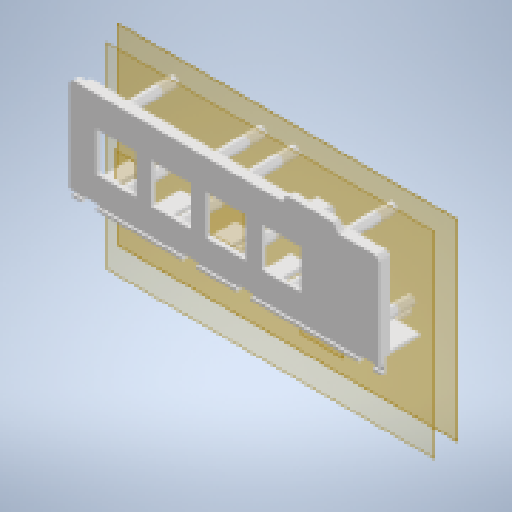
# Autodesk Inventor part: RV_ES_TopHV
Saved by Autodesk Inventor 2024.2 (Build 282272000, 272)
## iProperties
Created: 2023-08-06
Part Number: RV_ES_TopHV
Material: Generic
Document SubType Name: Modeling
Designer: atrus
Density: 1 g/cm^3
Appearance: Default
Mass: 78.5507 g
Surface Area: 462.891 cm^2
Volume: 78.5507 cm^3
Author: atrus
Autodesk Inventor part; units mm, degrees
ref_plane "YZ Plane" through (0, 0, 0) normal (1, 0, 0) x (0, 1, 0)
ref_plane "XZ Plane" through (0, 0, 0) normal (0, 1, 0) x (-1, 0, 0)
ref_plane "Work Plane1" through (160.7185, -7.942384, -39.091557) normal (0, 0, 1) x (1, 0, 0)
ref_plane "Bottom Case Offset" through (160.7185, -7.942384, -38.891557) normal (0, 0, 1) x (1, 0, 0)
sketch "Sketch1" plane through (0, 0, 0) normal (0, 0, 1) x (1, 0, 0)
  line L0 (0, 55.614096) -> (215.9, 55.614096)
  line L1 (215.9, 55.614096) -> (215.9, 121.724616)
  line L2 (215.9, 121.724616) -> (0, 121.724616)
  line L3 (0, 121.724616) -> (0, 55.614096)
  line L4 (215.9, 121.724616) -> (215.9, 57.656276) construction
  line L5 (0, 48.884616) -> (0, 118.549616)
  line L6 (1.113, 48.884616) -> (0, 48.884616)
  point P0 (0, 88.669356)
  constraints: 10 end point, 2 parallel, 1 horizontal, 1 midpoint, 1 perpendicular
extrude "Top Face" add sketch "Sketch1" along normal blind 5
sketch "Sketch2" plane through (0, 0, 5) normal (0, 0, 1) x (1, 0, 0)
  line L0 (44.754719, 74.175735) -> (19.253119, 74.175735) construction
  line L1 (44.754719, 99.677335) -> (44.754719, 74.175735) construction
  line L2 (19.253119, 74.175735) -> (19.253119, 99.677335) construction
  line L3 (57.607119, 74.175735) -> (57.607119, 99.677335) construction
  line L4 (83.108719, 99.677335) -> (83.108719, 74.175735) construction
  line L5 (83.108719, 74.175735) -> (57.607119, 74.175735) construction
  line L6 (96.215119, 74.175735) -> (96.215119, 99.677335) construction
  line L7 (121.716719, 99.677335) -> (121.716719, 74.175735) construction
  line L8 (134.823119, 74.175735) -> (134.823119, 99.677335) construction
  line L9 (160.324719, 99.677335) -> (160.324719, 74.175735) construction
  line L10 (160.324719, 74.175735) -> (134.823119, 74.175735) construction
  line L11 (19.253119, 99.677335) -> (44.754719, 99.677335) construction
  line L12 (57.607119, 99.677335) -> (83.108719, 99.677335) construction
  line L13 (96.215119, 99.677335) -> (121.716719, 99.677335) construction
  line L14 (134.823119, 99.677335) -> (160.324719, 99.677335) construction
  line L15 (18.253119, 100.677335) -> (18.253119, 73.175735)
  line L16 (18.253119, 73.175735) -> (45.754719, 73.175735)
  line L17 (45.754719, 73.175735) -> (45.754719, 100.677335)
  line L18 (45.754719, 100.677335) -> (18.253119, 100.677335)
  line L19 (56.607119, 100.677335) -> (56.607119, 73.175735)
  line L20 (56.607119, 73.175735) -> (84.108719, 73.175735)
  line L21 (84.108719, 73.175735) -> (84.108719, 100.677335)
  line L22 (84.108719, 100.677335) -> (56.607119, 100.677335)
  line L23 (121.716719, 74.175735) -> (96.215119, 74.175735) construction
  line L24 (96.215119, 74.175735) -> (96.215119, 99.677335)
  line L25 (95.215119, 100.677335) -> (95.215119, 73.175735)
  line L26 (95.215119, 73.175735) -> (122.716719, 73.175735)
  line L27 (122.716719, 73.175735) -> (122.716719, 100.677335)
  line L28 (122.716719, 100.677335) -> (95.215119, 100.677335)
  line L29 (133.823119, 100.677335) -> (133.823119, 73.175735)
  line L30 (133.823119, 73.175735) -> (161.324719, 73.175735)
  line L31 (161.324719, 73.175735) -> (161.324719, 100.677335)
  line L32 (161.324719, 100.677335) -> (133.823119, 100.677335)
  point P0 (0, 0)
  dimension "d96" = 1
  constraints: 32 end point, 3 parallel, 12 other
  measures "d96" distance between parallel lines of L18 L11
extrude "Recept Cutouts" cut sketch "Sketch2" against normal blind 3
sketch "Sketch3" plane through (0, 0, 0) normal (0, 0, -1) x (-1, 0, 0)
  circle A0 centre (-90.17, 112.834616) radius 3.750005 construction
  circle A1 centre (-181.61, 112.834616) radius 3.750005 construction
  circle A2 centre (-29.21, 112.834616) radius 3.550005
  circle A3 centre (-32.004, 65.844616) radius 3.550005
  circle A4 centre (-70.358, 65.844616) radius 3.550005
  circle A5 centre (-90.17, 112.834616) radius 3.550005
  circle A6 centre (-113.03, 112.834616) radius 3.550005
  circle A7 centre (-108.966, 65.844616) radius 3.550005
  circle A8 centre (-181.61, 112.834616) radius 3.550005
  circle A9 centre (-194.31, 63.304616) radius 3.550005
  circle A10 centre (-29.21, 112.834616) radius 3.81
  circle A11 centre (-32.004, 65.844616) radius 3.81
  circle A12 centre (-113.03, 112.834616) radius 3.81
  circle A13 centre (-70.358, 65.844616) radius 3.81
  circle A14 centre (-108.966, 65.844616) radius 3.81
  circle A15 centre (-194.31, 63.304616) radius 3.81
  circle A16 centre (-147.574, 65.844616) radius 3.750005
  circle A17 centre (-147.574, 65.844616) radius 3.550005
  point P0 (0, 0)
  dimension "d5" = 0.2
  constraints: 9 centre point, 8 equal radius, 7 coincident
  measures "d5" radial gap between concentric circles of A1 A8
extrude "Bosses" add sketch "Sketch3" along normal up to surface (38.891557 mm away) contours A2 | A3 | A4 | A5 | A6 | A7 | A8 | A9 | A17
ref_plane "PCB Plane Offset" through (103.01683, 55.15644, -27.328797) normal (0, 0, 1) x (1, 0, 0)
sketch "Sketch4" plane through (0, 0, 0) normal (0, 0, -1) x (-1, 0, 0)
  line L0 (-188.196091, 44.678615) -> (-188.196091, 97.078617) construction
  line L1 (-188.696091, 55.614096) -> (-212.089995, 55.614096)
  line L2 (-212.089995, 55.614096) -> (-212.089995, 57.846616)
  line L3 (-212.089995, 57.846616) -> (-188.696091, 57.846616)
  line L4 (-188.696091, 57.846616) -> (-188.696091, 55.614096)
  line L5 (-172.95, 57.946616) -> (-195.35, 57.946616)
  line L6 (-212.08999, -4.005394) -> (-212.09, 115.374616)
  line L7 (0, 55.614096) -> (-215.9, 55.614096)
  point P0 (0, 0)
  dimension "d8" = 0.5
  dimension "d109" = 0.1
  constraints: 8 end point, 3 perpendicular, 1 collinear, 1 horizontal
  measures "d8" distance between parallel lines of L0 L4
  measures "d109" distance between parallel lines of L5 L3
extrude "PS Side Tall Barrier" add sketch "Sketch4" along normal up to surface (27.328797 mm away)
sketch "Sketch5" plane through (212.089995, 57.846616, -27.328797) normal (0, 0, -1) x (-1, 0, 0)
  line L0 (23.393904, 0) -> (23.393904, -2.23252)
  line L1 (23.393904, 0) -> (0, 0)
  line L2 (23.393904, -2.23252) -> (16.939975, -2.23252)
  line L3 (16.939975, -2.23252) -> (16.939975, 0)
  line L4 (16.939975, 0) -> (23.393904, 0)
  line L5 (23.393904, 0) -> (23.393904, -2.23252)
  point P0 (212.089995, -57.846616)
  point P1 (16.739975, -2.8)
  dimension "d13" = 0.2
  constraints: 8 end point, 2 parallel, 1 horizontal, 1 perpendicular, 1 point on line, 1 other
  measures "d13" horizontal distance of point (16.74, -2.8) L2.end
extrude "PS Side Tall Barrier PCB" add sketch "Sketch5" along normal up to surface (11.56276 mm away)
sketch "Sketch6" plane through (0, 0, 0) normal (0, 0, -1) x (-1, 0, 0)
  arc A0 (-212.725, 121.724616) -> (-215.9, 118.549616) centre (-212.725, 118.549616) ccw construction
  arc A1 (-210.312, 119.311616) -> (-213.487, 116.136616) centre (-210.312, 116.136616) ccw construction
  line L0 (-213.487, 50.884616) -> (-213.487, 116.136616) construction
  line L1 (-210.312, 119.311616) -> (-172.72, 119.311616) construction
  line L2 (-162.72, 119.311616) -> (-5.588, 119.311616) construction
  arc A2 (-2.413, 116.136616) -> (-5.588, 119.311616) centre (-5.588, 116.136616) ccw construction
  line L3 (-2.413, 116.136616) -> (-2.413, 60.364616) construction
  line L4 (-213.287, 58.146616) -> (-213.287, 116.136616)
  arc A3 (-210.312, 119.111616) -> (-213.287, 116.136616) centre (-210.312, 116.136616) ccw
  line L5 (-210.312, 119.111616) -> (-172.72, 119.111616)
  line L6 (-162.72, 119.111616) -> (-5.588, 119.111616)
  arc A4 (-2.613, 116.136616) -> (-5.588, 119.111616) centre (-5.588, 116.136616) ccw
  line L7 (-2.613, 116.136616) -> (-2.613, 61.064616)
  line L8 (-211.287, 58.146616) -> (-211.287, 116.136616)
  arc A5 (-210.312, 117.111616) -> (-211.287, 116.136616) centre (-210.312, 116.136616) ccw
  arc A6 (-4.613, 116.136616) -> (-5.588, 117.111616) centre (-5.588, 116.136616) ccw
  line L9 (-4.613, 116.136616) -> (-4.613, 61.064616)
  line L10 (-211.287, 58.146616) -> (-213.287, 58.146616)
  line L11 (-4.613, 61.064616) -> (-2.613, 61.064616)
  line L12 (-162.72, 119.111616) -> (-162.72, 117.111616)
  line L13 (-172.72, 117.111616) -> (-172.72, 119.111616)
  circle A7 centre (-181.61, 112.834616) radius 3.550005
  line L14 (-178.059995, 112.834616) -> (-178.059995, 117.111616)
  circle A8 centre (-113.03, 112.834616) radius 3.550005
  line L15 (-116.580005, 112.834616) -> (-116.580005, 117.111616)
  line L16 (-109.479995, 112.834616) -> (-109.479995, 117.111616)
  circle A9 centre (-90.17, 112.834616) radius 3.550005
  line L17 (-93.720005, 112.834616) -> (-93.720005, 117.111616)
  line L18 (-86.619995, 112.834616) -> (-86.619995, 117.111616)
  circle A10 centre (-29.21, 112.834616) radius 3.550005
  line L19 (-32.760005, 112.834616) -> (-32.760005, 117.111616)
  line L20 (-25.659995, 112.834616) -> (-25.659995, 117.111616)
  circle A11 centre (-181.61, 112.834616) radius 3.550005
  circle A12 centre (-113.03, 112.834616) radius 3.550005
  line L21 (-185.160005, 112.834616) -> (-185.160005, 117.111616)
  line L22 (-210.312, 117.111616) -> (-185.160005, 117.111616)
  line L23 (-178.059995, 117.111616) -> (-172.72, 117.111616)
  line L24 (-162.72, 117.111616) -> (-116.580005, 117.111616)
  line L25 (-109.479995, 117.111616) -> (-93.720005, 117.111616)
  line L26 (-86.619995, 117.111616) -> (-32.760005, 117.111616)
  line L27 (-25.659995, 117.111616) -> (-5.588, 117.111616)
  line L28 (-195.15002, 57.846616) -> (-212.089995, 57.846616)
  line L29 (-3.81001, 60.764616) -> (-8.88109, 60.764616) construction
  line L30 (-188.696091, 57.846616) -> (-195.15002, 57.846616) construction
  point P0 (-212.287, 58.146616)
  dimension "d59" = 0.2
  dimension "d60" = 0.2
  dimension "d62" = 2
  dimension "d113" = 2
  dimension "d114" = 0.3
  dimension "d115" = 0.3
  constraints: 48 end point, 24 perpendicular, 15 point on circle, 8 collinear, 7 tangent, 4 centre point, 3 vertical, 2 horizontal, 2 parallel, 1 midpoint, 8 other
  measures "d59" distance between parallel lines of L2 L6
  measures "d60" distance between parallel lines of L0 L4
  measures "d62" distance of L13.start L5.end
  measures "d113" distance between parallel lines of L8 L4
  measures "d114" distance between parallel lines of L29 L11
  measures "d115" distance from line of L30 point (-212.287, 58.147)
extrude "Inner Lip" add sketch "Sketch6" along normal blind 5 contours L4 A3 L5 L13 L23 L14 A7 L21 L22 A5 L8 L10 | L6 A4 L7 L11 L9 A6 L27 L20 A10 L19 L26 L18 A9 L17 L25 L16 A8 L15 L24 L12
sketch "Sketch7" plane through (181.61, 112.834616, -38.891557) normal (0, 0, -1) x (-1, 0, 0)
  circle A0 centre (0, 0) radius 3.550005
  circle A1 centre (68.58, 0) radius 3.550005
  circle A2 centre (91.44, 0) radius 3.550005
  circle A3 centre (152.4, 0) radius 3.550005
  circle A4 centre (149.606, -46.99) radius 3.550005
  circle A5 centre (111.252, -46.99) radius 3.550005
  circle A6 centre (72.644, -46.99) radius 3.550005
  circle A7 centre (-12.7, -49.53) radius 3.550005
  circle A8 centre (34.036, -46.99) radius 3.550005
  point P0 (181.61, -112.834616)
hole "Boss Holes" at (181.61, 112.834616, -38.891557) at (113.03, 112.834616, -38.891557) at (90.17, 112.834616, -38.891557) at (29.21, 112.834616, -38.891557) at (32.004, 65.844616, -38.891557) at (70.358, 65.844616, -38.891557) at (108.966, 65.844616, -38.891557) at (194.31, 63.304616, -38.891557) at (147.574, 65.844616, -38.891557) direction (0, 0, 1) diameter 2.15646 depth 12.7 tip angle 118 thread size "4-40 UNC" class "2B" standard "ANSI Unified Screw Threads"
sketch "Sketch8" plane through (0, 0, 0) normal (0, 0, -1) x (-1, 0, 0)
  line L0 (-162.72, 117.111616) -> (-162.72, 121.724616)
  line L1 (-215.9, 121.724616) -> (0, 121.724616)
  line L2 (-172.72, 117.111616) -> (-172.72, 121.724616)
  line L3 (-162.72, 117.111616) -> (-116.580005, 117.111616) construction
  line L4 (-172.72, 117.111616) -> (-162.72, 117.111616)
  line L5 (-178.059995, 117.111616) -> (-172.72, 117.111616)
  line L6 (-172.72, 117.111616) -> (-172.72, 119.111616)
  line L7 (-162.72, 119.111616) -> (-162.72, 117.111616)
  line L8 (-172.72, 121.724616) -> (-162.72, 121.724616)
  point P0 (0, 0)
  point P1 (-172.72, 118.111616)
  constraints: 8 end point, 3 collinear, 1 horizontal, 1 midpoint, 1 perpendicular, 1 point on line, 1 vertical
extrude "Cord Relief" add sketch "Sketch8" along normal blind 7
fillet "Boss Filets" radius 3.175 9 edges at (181.61, 109.2846, 0) (35.554, 65.8446, 0) (73.908, 65.8446, 0) (112.516, 65.8446, 0) (197.86, 63.3046, 0) (113.03, 109.2846, 0) (90.17, 109.2846, 0) (29.21, 109.2846, 0) (151.124, 65.8446, 0)
ref_plane "Relay Top" through (28.37801, 48.104546, -10.841317) normal (0, 0, 1) x (0, -1, 0)
ref_plane "PS Top" through (155.310019, 43.098635, -2.554097) normal (0, 0, 1) x (0, 1, 0)
ref_plane "Work Plane7" through (-216.350226, -15.116245, -29.091557) normal (0, 0, 1) x (1, -0.0000001, 0)
sketch "Sketch10" plane through (0, 0, 0) normal (0, 0, -1) x (-1, 0, 0)
  line L0 (-160.996089, 97.078617) -> (-160.996089, 44.678615) construction
  line L1 (-188.196091, 44.678615) -> (-188.196091, 97.078617) construction
  line L2 (-122.08008, 67.154546) -> (-134.78008, 67.154546) construction
  line L3 (-134.78008, 67.154546) -> (-134.78008, 96.154546) construction
  line L4 (-134.78008, 96.154546) -> (-122.08008, 96.154546) construction
  line L5 (-122.08008, 96.154546) -> (-122.08008, 67.154546) construction
  line L6 (-123.43008, 68.054546) -> (-133.43008, 68.054546) construction
  line L7 (-123.43008, 69.054546) -> (-123.43008, 68.054546) construction
  line L8 (-133.43008, 69.054546) -> (-123.43008, 69.054546) construction
  line L9 (-133.43008, 68.054546) -> (-133.43008, 69.054546) construction
  line L10 (-133.83008, 88.254546) -> (-133.83008, 84.654546) construction
  line L11 (-133.83008, 84.654546) -> (-123.03008, 84.654546) construction
  line L12 (-123.03008, 84.654546) -> (-123.03008, 88.254546) construction
  line L13 (-123.03008, 88.254546) -> (-133.83008, 88.254546) construction
  line L14 (-83.21808, 67.154556) -> (-95.91808, 67.154556) construction
  line L15 (-95.91808, 67.154556) -> (-95.91808, 96.154556) construction
  line L16 (-95.91808, 96.154556) -> (-83.21808, 96.154556) construction
  line L17 (-83.21808, 96.154556) -> (-83.21808, 67.154556) construction
  line L18 (-84.56808, 68.054556) -> (-94.56808, 68.054556) construction
  line L19 (-84.56808, 69.054556) -> (-84.56808, 68.054556) construction
  line L20 (-94.56808, 69.054556) -> (-84.56808, 69.054556) construction
  line L21 (-94.56808, 68.054556) -> (-94.56808, 69.054556) construction
  line L22 (-94.96808, 88.254556) -> (-94.96808, 84.654556) construction
  line L23 (-94.96808, 84.654556) -> (-84.16808, 84.654556) construction
  line L24 (-84.16808, 84.654556) -> (-84.16808, 88.254556) construction
  line L25 (-84.16808, 88.254556) -> (-94.96808, 88.254556) construction
  line L26 (-44.86408, 67.154546) -> (-57.56408, 67.154546) construction
  line L27 (-57.56408, 67.154546) -> (-57.56408, 96.154546) construction
  line L28 (-57.56408, 96.154546) -> (-44.86408, 96.154546) construction
  line L29 (-44.86408, 96.154546) -> (-44.86408, 67.154546) construction
  line L30 (-46.21408, 68.054546) -> (-56.21408, 68.054546) construction
  line L31 (-46.21408, 69.054546) -> (-46.21408, 68.054546) construction
  line L32 (-56.21408, 69.054546) -> (-46.21408, 69.054546) construction
  line L33 (-56.21408, 68.054546) -> (-56.21408, 69.054546) construction
  line L34 (-56.61408, 88.254546) -> (-56.61408, 84.654546) construction
  line L35 (-56.61408, 84.654546) -> (-45.81408, 84.654546) construction
  line L36 (-45.81408, 84.654546) -> (-45.81408, 88.254546) construction
  line L37 (-45.81408, 88.254546) -> (-56.61408, 88.254546) construction
  line L38 (-6.13608, 67.154546) -> (-18.83608, 67.154546) construction
  line L39 (-18.83608, 67.154546) -> (-18.83608, 96.154546) construction
  line L40 (-18.83608, 96.154546) -> (-6.13608, 96.154546) construction
  line L41 (-6.13608, 96.154546) -> (-6.13608, 67.154546) construction
  line L42 (-7.48608, 68.054546) -> (-17.48608, 68.054546) construction
  line L43 (-7.48608, 69.054546) -> (-7.48608, 68.054546) construction
  line L44 (-17.48608, 69.054546) -> (-7.48608, 69.054546) construction
  line L45 (-17.48608, 68.054546) -> (-17.48608, 69.054546) construction
  line L46 (-17.88608, 88.254546) -> (-17.88608, 84.654546) construction
  line L47 (-17.88608, 84.654546) -> (-7.08608, 84.654546) construction
  line L48 (-7.08608, 84.654546) -> (-7.08608, 88.254546) construction
  line L49 (-7.08608, 88.254546) -> (-17.88608, 88.254546) construction
  line L50 (-195.15002, 55.614096) -> (-188.696091, 55.614096)
  line L51 (-188.696091, 55.614096) -> (-188.696091, 57.846616)
  line L52 (-188.696091, 57.846616) -> (-195.15002, 57.846616)
  line L53 (-195.15002, 57.846616) -> (-195.15002, 55.614096)
  line L54 (0, 55.614096) -> (-215.9, 55.614096)
  line L55 (-188.696091, 57.846616) -> (-195.15002, 57.846616)
  arc A0 (-43.204, 60.994616) -> (-43.204, 57.994616) centre (-43.204, 59.494616) ccw construction
  arc A1 (-59.158, 57.994616) -> (-59.158, 60.994616) centre (-59.158, 59.494616) ccw construction
  arc A2 (-81.558, 60.994616) -> (-81.558, 57.994616) centre (-81.558, 59.494616) ccw construction
  arc A3 (-97.766, 57.994616) -> (-97.766, 60.994616) centre (-97.766, 59.494616) ccw construction
  arc A4 (-120.166, 60.994616) -> (-120.166, 57.994616) centre (-120.166, 59.494616) ccw construction
  arc A5 (-135.358, 57.994616) -> (-135.358, 60.994616) centre (-135.358, 59.494616) ccw construction
  arc A6 (-157.758, 60.994616) -> (-157.758, 57.994616) centre (-157.758, 59.494616) ccw construction
  arc A7 (-20.804, 57.994616) -> (-20.804, 60.994616) centre (-20.804, 59.494616) ccw construction
  line L56 (-8.88109, 60.764616) -> (-8.88109, 58.224616) construction
  line L57 (-9.18109, 60.994616) -> (-19.004, 60.994616)
  line L58 (-19.004, 60.994616) -> (-19.004, 57.994616)
  line L59 (-19.004, 57.994616) -> (-9.18109, 57.994616)
  line L60 (-9.18109, 57.994616) -> (-9.18109, 60.994616)
  line L61 (-20.804, 57.994616) -> (-8.060378, 57.994616) construction
  line L62 (-20.804, 60.994616) -> (-8.354564, 60.994616) construction
  line L63 (-45.004, 60.994616) -> (-57.358, 60.994616)
  line L64 (-57.358, 60.994616) -> (-57.358, 57.994616)
  line L65 (-57.358, 57.994616) -> (-45.004, 57.994616)
  line L66 (-45.004, 57.994616) -> (-45.004, 60.994616)
  line L67 (-83.358, 57.994616) -> (-95.966, 57.994616)
  line L68 (-95.966, 57.994616) -> (-95.966, 60.994616)
  line L69 (-95.966, 60.994616) -> (-83.358, 60.994616)
  line L70 (-83.358, 60.994616) -> (-83.358, 57.994616)
  line L71 (-121.966, 57.994616) -> (-133.558, 57.994616)
  line L72 (-133.558, 57.994616) -> (-133.558, 60.994616)
  line L73 (-133.558, 60.994616) -> (-121.966, 60.994616)
  line L74 (-121.966, 60.994616) -> (-121.966, 57.994616)
  point P0 (-19.304, 59.494616)
  point P1 (-9.18109, 59.494616)
  point P2 (-45.004, 59.494616)
  point P3 (-44.704, 59.494616)
  point P4 (-57.658, 59.494616)
  point P5 (-57.358, 59.494616)
  point P6 (-83.358, 59.494616)
  point P7 (-83.058, 59.494616)
  point P8 (-96.266, 59.494616)
  point P9 (-95.966, 59.494616)
  point P10 (-121.666, 59.494616)
  point P11 (-121.966, 59.494616)
  point P12 (-133.858, 59.494616)
  point P13 (-133.558, 59.494616)
  dimension "d101" = 0.3
  dimension "d102" = 0.3
  dimension "d103" = 0.3
  dimension "d104" = 0.3
  dimension "d105" = 0.3
  dimension "d106" = 0.3
  dimension "d107" = 0.3
  dimension "d108" = 0.3
  constraints: 36 end point, 8 collinear, 8 parallel, 7 midpoint, 7 point on circle, 6 horizontal, 4 perpendicular
  measures "d101" distance from line of point (-19.304, 59.495) L58
  measures "d102" distance from line of point (-9.181, 59.495) L56
  measures "d103" distance of point (-45.004, 59.495) point (-44.704, 59.495)
  measures "d104" distance of point (-57.658, 59.495) point (-57.358, 59.495)
  measures "d105" distance of point (-83.358, 59.495) point (-83.058, 59.495)
  measures "d106" distance of point (-96.266, 59.495) point (-95.966, 59.495)
  measures "d107" distance of point (-121.666, 59.495) point (-121.966, 59.495)
  measures "d108" distance of point (-133.858, 59.495) point (-133.558, 59.495)
extrude "Barrier Relay" add sketch "Sketch10" along normal up to surface (27.328797 mm away) contours L60 L59 L58 L57 | L66 L65 L64 L63 | L67 L68 L69 L70 | L71 L72 L73 L74
sketch "Sketch11" plane through (0, 0, 0) normal (0, 0, -1) x (-1, 0, 0)
  line L0 (-160.996089, 97.078617) -> (-160.996089, 44.678615) construction
  line L1 (-188.196091, 44.678615) -> (-188.196091, 97.078617) construction
  line L2 (0, 55.614096) -> (-215.9, 55.614096)
  line L3 (-187.696091, 55.614096) -> (-161.496089, 55.614096)
  line L4 (-161.496089, 55.614096) -> (-161.496089, 57.846616)
  line L5 (-161.496089, 57.846616) -> (-187.696091, 57.846616)
  line L6 (-187.696091, 57.846616) -> (-187.696091, 55.614096)
  line L7 (-188.696091, 57.846616) -> (-195.15002, 57.846616) construction
  point P0 (0, 0)
  point P1 (-187.696091, 56.730356)
  point P2 (-161.496089, 56.730356)
  dimension "d55" = 0.5
  dimension "d56" = 0.5
  constraints: 8 end point, 2 midpoint, 2 parallel, 1 collinear, 1 horizontal, 1 perpendicular, 1 point on line
  measures "d55" distance from line of L1 point (-187.696, 56.73)
  measures "d56" distance from line of point (-161.496, 56.73) L0
extrude "Barrier PSU" add sketch "Sketch11" along normal up to surface (2.554097 mm away)
fillet "Outside corner fillets" radius 3.175 2 edges at (215.9, 121.7246, 2.5) (0, 121.7246, 2.5)
fillet "Outer Boss Fillets" radius 3.175 4 edges at (29.21, 116.3846, -5) (90.17, 116.3846, -5) (113.03, 116.3846, -5) (181.61, 116.3846, -5)
ref_plane "TopReceptSeatOffset" through (100.625339, 92.026755, 2.44) normal (0, 0, 1) x (-1, 0, 0)
sketch "Sketch12" plane through (0, 0, 0) normal (0, 0, -1) x (-1, 0, 0)
  line L0 (-20.408819, 71.369035) -> (-43.599019, 71.369035) construction
  arc A0 (-20.408819, 71.369035) -> (-16.446419, 75.331435) centre (-20.408819, 75.331435) ccw construction
  line L1 (-16.446419, 98.521635) -> (-16.446419, 75.331435) construction
  arc A1 (-16.446419, 98.521635) -> (-20.408819, 102.484035) centre (-20.408819, 98.521635) ccw construction
  line L2 (-43.599019, 102.484035) -> (-20.408819, 102.484035) construction
  arc A2 (-43.599019, 102.484035) -> (-47.561419, 98.521635) centre (-43.599019, 98.521635) ccw construction
  line L3 (-47.561419, 75.331435) -> (-47.561419, 98.521635) construction
  arc A3 (-47.561419, 75.331435) -> (-43.599019, 71.369035) centre (-43.599019, 75.331435) ccw construction
  line L4 (-43.167219, 74.975835) -> (-20.815219, 74.975835) construction
  arc A4 (-43.929219, 75.737835) -> (-43.167219, 74.975835) centre (-43.167219, 75.737835) ccw construction
  line L5 (-43.929219, 88.691835) -> (-43.929219, 75.737835) construction
  arc A5 (-43.167219, 89.453835) -> (-43.929219, 88.691835) centre (-43.167219, 88.691835) ccw construction
  line L6 (-40.385919, 89.453835) -> (-43.167219, 89.453835) construction
  arc A6 (-40.385919, 89.453835) -> (-39.623919, 90.215835) centre (-40.385919, 90.215835) ccw construction
  line L7 (-39.623919, 98.089835) -> (-39.623919, 90.215835) construction
  arc A7 (-38.861919, 98.851835) -> (-39.623919, 98.089835) centre (-38.861919, 98.089835) ccw construction
  line L8 (-25.145919, 98.851835) -> (-38.861919, 98.851835) construction
  arc A8 (-24.383919, 98.089835) -> (-25.145919, 98.851835) centre (-25.145919, 98.089835) ccw construction
  line L9 (-24.383919, 90.215835) -> (-24.383919, 98.089835) construction
  arc A9 (-24.383919, 90.215835) -> (-23.621919, 89.453835) centre (-23.621919, 90.215835) ccw construction
  line L10 (-20.815219, 89.453835) -> (-23.621919, 89.453835) construction
  arc A10 (-20.053219, 88.691835) -> (-20.815219, 89.453835) centre (-20.815219, 88.691835) ccw construction
  line L11 (-20.053219, 75.737835) -> (-20.053219, 88.691835) construction
  arc A11 (-20.815219, 74.975835) -> (-20.053219, 75.737835) centre (-20.815219, 75.737835) ccw construction
  line L12 (-58.762819, 71.369035) -> (-81.953019, 71.369035) construction
  arc A12 (-58.762819, 71.369035) -> (-54.800419, 75.331435) centre (-58.762819, 75.331435) ccw construction
  line L13 (-54.800419, 98.521635) -> (-54.800419, 75.331435) construction
  arc A13 (-54.800419, 98.521635) -> (-58.762819, 102.484035) centre (-58.762819, 98.521635) ccw construction
  line L14 (-81.953019, 102.484035) -> (-58.762819, 102.484035) construction
  arc A14 (-81.953019, 102.484035) -> (-85.915419, 98.521635) centre (-81.953019, 98.521635) ccw construction
  line L15 (-85.915419, 75.331435) -> (-85.915419, 98.521635) construction
  arc A15 (-85.915419, 75.331435) -> (-81.953019, 71.369035) centre (-81.953019, 75.331435) ccw construction
  line L16 (-81.521219, 74.975835) -> (-59.169219, 74.975835) construction
  arc A16 (-82.283219, 75.737835) -> (-81.521219, 74.975835) centre (-81.521219, 75.737835) ccw construction
  line L17 (-82.283219, 88.691835) -> (-82.283219, 75.737835) construction
  arc A17 (-81.521219, 89.453835) -> (-82.283219, 88.691835) centre (-81.521219, 88.691835) ccw construction
  line L18 (-78.739919, 89.453835) -> (-81.521219, 89.453835) construction
  arc A18 (-78.739919, 89.453835) -> (-77.977919, 90.215835) centre (-78.739919, 90.215835) ccw construction
  line L19 (-77.977919, 98.089835) -> (-77.977919, 90.215835) construction
  arc A19 (-77.215919, 98.851835) -> (-77.977919, 98.089835) centre (-77.215919, 98.089835) ccw construction
  line L20 (-63.499919, 98.851835) -> (-77.215919, 98.851835) construction
  arc A20 (-62.737919, 98.089835) -> (-63.499919, 98.851835) centre (-63.499919, 98.089835) ccw construction
  line L21 (-62.737919, 90.215835) -> (-62.737919, 98.089835) construction
  arc A21 (-62.737919, 90.215835) -> (-61.975919, 89.453835) centre (-61.975919, 90.215835) ccw construction
  line L22 (-59.169219, 89.453835) -> (-61.975919, 89.453835) construction
  arc A22 (-58.407219, 88.691835) -> (-59.169219, 89.453835) centre (-59.169219, 88.691835) ccw construction
  line L23 (-58.407219, 75.737835) -> (-58.407219, 88.691835) construction
  arc A23 (-59.169219, 74.975835) -> (-58.407219, 75.737835) centre (-59.169219, 75.737835) ccw construction
  line L24 (-124.523419, 75.331435) -> (-124.523419, 98.521635) construction
  arc A24 (-120.561019, 102.484035) -> (-124.523419, 98.521635) centre (-120.561019, 98.521635) ccw construction
  line L25 (-120.561019, 102.484035) -> (-97.370819, 102.484035) construction
  arc A25 (-93.408419, 98.521635) -> (-97.370819, 102.484035) centre (-97.370819, 98.521635) ccw construction
  line L26 (-93.408419, 98.521635) -> (-93.408419, 75.331435) construction
  arc A26 (-97.370819, 71.369035) -> (-93.408419, 75.331435) centre (-97.370819, 75.331435) ccw construction
  line L27 (-97.370819, 71.369035) -> (-120.561019, 71.369035) construction
  arc A27 (-124.523419, 75.331435) -> (-120.561019, 71.369035) centre (-120.561019, 75.331435) ccw construction
  line L28 (-96.215119, 74.175735) -> (-121.716719, 74.175735) construction
  line L29 (-96.215119, 99.677335) -> (-96.215119, 74.175735) construction
  line L30 (-121.716719, 99.677335) -> (-96.215119, 99.677335) construction
  line L31 (-121.716719, 74.175735) -> (-121.716719, 99.677335) construction
  line L32 (-135.978819, 71.369035) -> (-159.169019, 71.369035) construction
  arc A28 (-135.978819, 71.369035) -> (-132.016419, 75.331435) centre (-135.978819, 75.331435) ccw construction
  line L33 (-132.016419, 98.521635) -> (-132.016419, 75.331435) construction
  arc A29 (-132.016419, 98.521635) -> (-135.978819, 102.484035) centre (-135.978819, 98.521635) ccw construction
  line L34 (-159.169019, 102.484035) -> (-135.978819, 102.484035) construction
  arc A30 (-159.169019, 102.484035) -> (-163.131419, 98.521635) centre (-159.169019, 98.521635) ccw construction
  line L35 (-163.131419, 75.331435) -> (-163.131419, 98.521635) construction
  arc A31 (-163.131419, 75.331435) -> (-159.169019, 71.369035) centre (-159.169019, 75.331435) ccw construction
  arc A32 (-58.762819, 75.331415) -> (-58.762799, 75.331435) centre (-58.762819, 75.331435) ccw
  arc A33 (-81.953038, 75.331435) -> (-81.953019, 75.331415) centre (-81.953019, 75.331435) ccw
  arc A34 (-81.953019, 98.521654) -> (-81.953038, 98.521635) centre (-81.953019, 98.521635) ccw
  arc A35 (-58.762799, 98.521635) -> (-58.762819, 98.521654) centre (-58.762819, 98.521635) ccw
  arc A36 (-135.978819, 75.331239) -> (-135.978623, 75.331435) centre (-135.978819, 75.331435) ccw
  arc A37 (-159.169214, 75.331435) -> (-159.169019, 75.331239) centre (-159.169019, 75.331435) ccw
  arc A38 (-159.169019, 98.52183) -> (-159.169214, 98.521635) centre (-159.169019, 98.521635) ccw
  arc A39 (-135.978623, 98.521635) -> (-135.978819, 98.52183) centre (-135.978819, 98.521635) ccw
  arc A40 (-131.016419, 98.521635) -> (-135.978819, 103.484035) centre (-135.978819, 98.521635) ccw
  line L36 (-131.016419, 98.521635) -> (-131.016419, 75.331435)
  arc A41 (-135.978819, 70.369035) -> (-131.016419, 75.331435) centre (-135.978819, 75.331435) ccw
  line L37 (-135.978819, 70.369035) -> (-159.169019, 70.369035)
  arc A42 (-164.131419, 75.331435) -> (-159.169019, 70.369035) centre (-159.169019, 75.331435) ccw
  line L38 (-164.131419, 75.331435) -> (-164.131419, 98.521635)
  arc A43 (-159.169019, 103.484035) -> (-164.131419, 98.521635) centre (-159.169019, 98.521635) ccw
  line L39 (-159.169019, 103.484035) -> (-135.978819, 103.484035)
  line L40 (-97.370819, 103.484035) -> (-120.561019, 103.484035)
  arc A44 (-120.561019, 103.484035) -> (-125.523419, 98.521635) centre (-120.561019, 98.521635) ccw
  line L41 (-125.523419, 98.521635) -> (-125.523419, 75.331435)
  arc A45 (-125.523419, 75.331435) -> (-120.561019, 70.369035) centre (-120.561019, 75.331435) ccw
  line L42 (-120.561019, 70.369035) -> (-97.370819, 70.369035)
  arc A46 (-97.370819, 70.369035) -> (-92.408419, 75.331435) centre (-97.370819, 75.331435) ccw
  line L43 (-92.408419, 75.331435) -> (-92.408419, 98.521635)
  arc A47 (-92.408419, 98.521635) -> (-97.370819, 103.484035) centre (-97.370819, 98.521635) ccw
  arc A48 (-53.800419, 98.521635) -> (-58.762819, 103.484035) centre (-58.762819, 98.521635) ccw
  line L44 (-53.800419, 98.521635) -> (-53.800419, 75.331435)
  arc A49 (-58.762819, 70.369035) -> (-53.800419, 75.331435) centre (-58.762819, 75.331435) ccw
  line L45 (-58.762819, 70.369035) -> (-81.953019, 70.369035)
  arc A50 (-86.915419, 75.331435) -> (-81.953019, 70.369035) centre (-81.953019, 75.331435) ccw
  line L46 (-86.915419, 75.331435) -> (-86.915419, 98.521635)
  arc A51 (-81.953019, 103.484035) -> (-86.915419, 98.521635) centre (-81.953019, 98.521635) ccw
  line L47 (-81.953019, 103.484035) -> (-58.762819, 103.484035)
  arc A52 (-15.446419, 98.521635) -> (-20.408819, 103.484035) centre (-20.408819, 98.521635) ccw
  line L48 (-15.446419, 98.521635) -> (-15.446419, 75.331435)
  arc A53 (-20.408819, 70.369035) -> (-15.446419, 75.331435) centre (-20.408819, 75.331435) ccw
  line L49 (-20.408819, 70.369035) -> (-43.599019, 70.369035)
  arc A54 (-48.561419, 75.331435) -> (-43.599019, 70.369035) centre (-43.599019, 75.331435) ccw
  line L50 (-48.561419, 75.331435) -> (-48.561419, 98.521635)
  arc A55 (-43.599019, 103.484035) -> (-48.561419, 98.521635) centre (-43.599019, 98.521635) ccw
  line L51 (-43.599019, 103.484035) -> (-20.408819, 103.484035)
  point P0 (0, 0)
  dimension "d97" = 1
  dimension "d98" = 1
  dimension "d99" = 1
  dimension "d100" = 1
  constraints: 48 point on circle, 32 end point, 24 centre point, 28 other
  measures "d97" distance between parallel lines of L34 L39
  measures "d98" distance between parallel lines of L25 L40
  measures "d99" distance between parallel lines of L47 L14
  measures "d100" distance between parallel lines of L51 L2
extrude "Recept Inset" cut sketch "Sketch12" along normal blind 4 and the other way blind 2.0066 contours A36 | A37 | A38 | A39 | L36 A41 L37 A42 L38 A43 L39 A40 | A47 L43 A46 L42 A45 L41 A44 L40 | L44 A49 L45 A50 L46 A51 L47 A48 | L48 A53 L49 A54 L50 A55 L51 A52
sketch "Sketch13" plane through (0, 55.614096, 0) normal (-1, 0, 0) x (0, 0, 1)
  line L0 (0, 0) -> (-10.841317, 0)
  line L1 (0, 0) -> (5, 0)
  line L2 (0, 0) -> (5, 0)
  line L3 (0, -6.65) -> (0, 0)
  line L4 (0, 62.93552) -> (0, 0)
  line L5 (5, 0) -> (5, 62.93552)
  line L6 (5, 0) -> (5, 0)
  line L7 (4, -1) -> (1.5, -1)
  line L8 (1.5, -1) -> (1.5, -4.65)
  line L9 (1.5, -4.65) -> (3, -4.65)
  line L10 (3, -4.65) -> (3, -6.65)
  line L11 (3, -6.65) -> (0, -6.65)
  line L12 (5, 0) -> (4, -1)
  line L13 (-23.851557, -6.72948) -> (-0.1, -6.72948) construction
  line L14 (0, 0) -> (-10.841317, 0)
  line L15 (0, 0) -> (5, 0) construction
  line L16 (0, 0) -> (0, -7.071912) construction
  point P0 (0, -55.614096)
  point P1 (5, -1)
  point P2 (0, -3.325)
  point P3 (1.5, 0.07052)
  point P4 (1.5, 0)
  dimension "d73" = 2
  dimension "d74" = 1.5
  dimension "d75" = 1
  dimension "d77" = 1
  dimension "d78" = 1
  dimension "d110" = 2
  dimension "d111" = 3.65
  constraints: 24 end point, 5 perpendicular, 3 point on line, 2 vertical, 1 midpoint
  measures "d73" distance between parallel lines of L6 L10
  measures "d74" distance from line of point (0, -3.325) L8
  measures "d75" distance of L1.end point (5, -1)
  measures "d77" distance of L6.end point (5, -1)
  measures "d78" distance of L7.start point (5, -1)
  measures "d110" distance of L9.end L10.end
  measures "d111" distance of L7.end L8.end
extrude "TopFace Interlock" add sketch "Sketch13" against normal up to surface (215.9 mm away)
sketch "Sketch14" plane through (0, 0, 5) normal (0, 0, 1) x (1, 0, 0)
  line L0 (18.253119, 103.217335) -> (45.754719, 103.217335) construction
  line L1 (56.353119, 103.217335) -> (84.108719, 103.217335) construction
  line L2 (94.453119, 103.217335) -> (122.716719, 103.217335) construction
  line L3 (132.553119, 103.217335) -> (161.324719, 103.217335) construction
  line L4 (133.823119, 100.677335) -> (161.324719, 100.677335) construction
  line L5 (95.215119, 100.677335) -> (122.716719, 100.677335) construction
  line L6 (56.607119, 100.677335) -> (84.108719, 100.677335) construction
  line L7 (18.253119, 100.677335) -> (45.754719, 100.677335) construction
  spline S0 degree 2 poles (149.902252, 107.122926) (149.902252, 106.235292) (149.465263, 104.794593) (148.536661, 103.770399) (147.095962, 103.217335) (146.085424, 103.217335) knots 0 0 0 1 2 3 4 4 4
  line L8 (146.085424, 103.217335) -> (144.153112, 103.217335)
  line L9 (144.153112, 103.217335) -> (144.153112, 110.837335)
  line L10 (144.153112, 110.837335) -> (146.406338, 110.837335)
  spline S1 degree 2 poles (146.406338, 110.837335) (147.280316, 110.837335) (148.591284, 110.400346) (149.465263, 109.492227) (149.902252, 108.092496) (149.902252, 107.122926) knots 0 0 0 1 2 3 4 4 4
  spline S2 degree 2 poles (148.365962, 107.027335) (148.365962, 107.648679) (148.167951, 108.618249) (147.696822, 109.287388) (146.904779, 109.635614) (146.317575, 109.635614) knots 0 0 0 1 2 3 4 4 4
  line L11 (146.317575, 109.635614) -> (145.586983, 109.635614)
  line L12 (145.586983, 109.635614) -> (145.586983, 104.419055)
  line L13 (145.586983, 104.419055) -> (146.215155, 104.419055)
  spline S3 degree 2 poles (146.215155, 104.419055) (147.273489, 104.419055) (148.365962, 105.675399) (148.365962, 107.027335) knots 0 0 0 1 2 2 2
  spline S4 degree 2 poles (111.152231, 103.524593) (110.646962, 103.319754) (109.697876, 103.114915) (109.178951, 103.114915) knots 0 0 0 1 2 2 2
  spline S5 degree 2 poles (109.178951, 103.114915) (108.359596, 103.114915) (107.096424, 103.5997) (106.229273, 104.555614) (105.778628, 105.969001) (105.778628, 106.911259) knots 0 0 0 1 2 3 4 4 4
  spline S6 degree 2 poles (105.778628, 106.911259) (105.778628, 107.874001) (106.270241, 109.369324) (107.178359, 110.407173) (108.475671, 110.946582) (109.288198, 110.946582) knots 0 0 0 1 2 3 4 4 4
  spline S7 degree 2 poles (109.288198, 110.946582) (109.547661, 110.946582) (110.011962, 110.926098) (110.455779, 110.857819) (110.906424, 110.755399) (111.152231, 110.673464) knots 0 0 0 1 2 3 4 4 4
  line L14 (111.152231, 110.673464) -> (111.152231, 109.253249)
  spline S8 degree 2 poles (111.152231, 109.253249) (110.660618, 109.485399) (109.759327, 109.68341) (109.390618, 109.68341) knots 0 0 0 1 2 2 2
  spline S9 degree 2 poles (109.390618, 109.68341) (108.851209, 109.68341) (108.086478, 109.294216) (107.588037, 108.584109) (107.355886, 107.614539) (107.355886, 107.027335) knots 0 0 0 1 2 3 4 4 4
  spline S10 degree 2 poles (107.355886, 107.027335) (107.355886, 106.412818) (107.594865, 105.436421) (108.093306, 104.760453) (108.878521, 104.405399) (109.411101, 104.405399) knots 0 0 0 1 2 3 4 4 4
  spline S11 degree 2 poles (109.411101, 104.405399) (109.602284, 104.405399) (110.052929, 104.480507) (110.510403, 104.60341) (110.961048, 104.774109) (111.152231, 104.862872) knots 0 0 0 1 2 3 4 4 4
  line L15 (111.152231, 104.862872) -> (111.152231, 103.524593)
  line L16 (67.697746, 103.217335) -> (67.697746, 110.837335)
  line L17 (67.697746, 110.837335) -> (70.155811, 110.837335)
  spline S12 degree 2 poles (70.155811, 110.837335) (71.459951, 110.837335) (72.757263, 109.929216) (72.757263, 109.007442) knots 0 0 0 1 2 2 2
  spline S13 degree 2 poles (72.757263, 109.007442) (72.757263, 108.727496) (72.620704, 108.181259) (72.340757, 107.730614) (71.924252, 107.382388) (71.637478, 107.279969) knots 0 0 0 1 2 3 4 4 4
  spline S14 degree 2 poles (71.637478, 107.279969) (71.924252, 107.232173) (72.443177, 106.959055) (72.83237, 106.522066) (73.057693, 105.928034) (73.057693, 105.559324) knots 0 0 0 1 2 3 4 4 4
  spline S15 degree 2 poles (73.057693, 105.559324) (73.057693, 104.391743) (71.494091, 103.217335) (70.019252, 103.217335) knots 0 0 0 1 2 2 2
  line L18 (70.019252, 103.217335) -> (67.697746, 103.217335)
  spline S16 degree 2 poles (70.121671, 104.391743) (70.463069, 104.391743) (70.981994, 104.56927) (71.337048, 104.876528) (71.514575, 105.293034) (71.514575, 105.532012) knots 0 0 0 1 2 3 4 4 4
  spline S17 degree 2 poles (71.514575, 105.532012) (71.514575, 106.030453) (70.777155, 106.590345) (70.012424, 106.590345) knots 0 0 0 1 2 2 2
  line L19 (70.012424, 106.590345) -> (69.117962, 106.590345)
  line L20 (69.117962, 106.590345) -> (69.117962, 104.391743)
  line L21 (69.117962, 104.391743) -> (70.121671, 104.391743)
  spline S18 degree 2 poles (71.26194, 108.754808) (71.26194, 108.973302) (71.125381, 109.321528) (70.811295, 109.560507) (70.32651, 109.697066) (69.985112, 109.697066) knots 0 0 0 1 2 3 4 4 4
  line L22 (69.985112, 109.697066) -> (69.117962, 109.697066)
  line L23 (69.117962, 109.697066) -> (69.117962, 107.689646)
  line L24 (69.117962, 107.689646) -> (69.985112, 107.689646)
  spline S19 degree 2 poles (69.985112, 107.689646) (70.333338, 107.689646) (70.818123, 107.860345) (71.125381, 108.153948) (71.26194, 108.536313) (71.26194, 108.754808) knots 0 0 0 1 2 3 4 4 4
  line L25 (33.676768, 103.217335) -> (33.260263, 104.719485)
  line L26 (33.260263, 104.719485) -> (30.597359, 104.719485)
  line L27 (30.597359, 104.719485) -> (30.167198, 103.217335)
  line L28 (30.167198, 103.217335) -> (28.746983, 103.217335)
  line L29 (28.746983, 103.217335) -> (31.000209, 110.837335)
  line L30 (31.000209, 110.837335) -> (33.007628, 110.837335)
  line L31 (33.007628, 110.837335) -> (35.267682, 103.217335)
  line L32 (35.267682, 103.217335) -> (33.676768, 103.217335)
  line L33 (31.949295, 109.444431) -> (30.938757, 105.893894)
  line L34 (30.938757, 105.893894) -> (32.932521, 105.893894)
  line L35 (32.932521, 105.893894) -> (31.949295, 109.444431)
  point P0 (0, 0)
  dimension "d112" = 2.54
  constraints: 8 end point, 4 horizontal, 4 vertical alignment, 3 collinear
  measures "d112" distance between parallel lines of L4 L3
extrude "Extrusion13" cut sketch "Sketch14" against normal blind 0.001
sketch "Sketch16" plane through (0, 0, 0) normal (0, 0, -1) x (-1, 0, 0)
  circle A0 centre (-204.47, 50.604616) radius 3.450005 construction
  circle A1 centre (-204.47, 50.604616) radius 4.99402
  line L0 (-212.089995, 55.598636) -> (-188.696091, 55.598636)
  circle A2 centre (-119.38, 50.604616) radius 3.450005 construction
  circle A3 centre (-81.28, 50.604616) radius 3.450005 construction
  circle A4 centre (-11.43, 50.604616) radius 3.450005 construction
  circle A5 centre (-119.38, 50.604616) radius 5.00948
  line L1 (0, 55.614096) -> (-215.9, 55.614096) construction
  circle A6 centre (-81.28, 50.604616) radius 5.00948
  circle A7 centre (-11.43, 50.604616) radius 5.00948
  point P0 (0, 0)
  constraints: 4 centre point, 4 coincident, 4 tangent
extrude "Extrusion14" cut sketch "Sketch16" against normal blind 25.4
sketch "Sketch17" plane through (0, 0, 0) normal (0, 0, -1) x (-1, 0, 0)
  line L0 (-212.725, 121.724616) -> (-172.72, 121.724616)
  line L1 (-162.72, 121.724616) -> (-172.72, 121.724616)
  line L2 (-162.72, 121.724616) -> (-3.175, 121.724616)
  line L3 (-153.059104, 126.804616) -> (-182.373296, 126.804616)
  arc A0 (-182.373296, 126.804616) -> (-185.484148, 124.264616) centre (-182.373296, 123.629616) ccw
  arc A1 (-188.595, 121.724616) -> (-185.484148, 124.264616) centre (-188.595, 124.899616) ccw
  arc A2 (-149.948252, 124.264616) -> (-153.059104, 126.804616) centre (-153.059104, 123.629616) ccw
  arc A3 (-149.948252, 124.264616) -> (-146.8374, 121.724616) centre (-146.8374, 124.899616) ccw
  point P0 (0, 0)
extrude "Extrusion15" add sketch "Sketch17" against normal up to surface (5 mm away)
sketch "Sketch18" plane through (162.72, 121.724616, 0) normal (0, 1, 0) x (1, 0, 0)
  line L0 (0, 0) -> (10, 0) projected
  line L1 (10, 0) -> (10, 7) projected
  line L2 (0, 7) -> (10, 7) projected
  line L3 (0, 0) -> (0, 7) projected
  point P0 (-162.72, 0)
extrude "Extrusion16" add sketch "Sketch18" along normal up to surface (5.08 mm away)
fillet "Fillet5" radius 3.175 1 edges at (167.72, 126.8046, -7)
equation "\"d78\" = d77"
body "Solid1"
